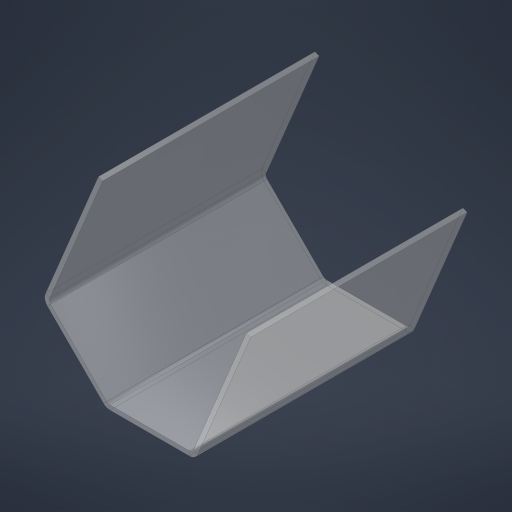
# Autodesk Inventor part: GP3-002
Saved by Autodesk Inventor 2023.4 (Build 274418000, 418)
## iProperties
Created: 2025-01-14
Part Number: GP3-002
Material: Polycarbonate, Clear
Document SubType Name: Sheet Metal
Designer: brand
Density: 1.2 g/cm^3
Sheet Metal Rule: Default
Appearance: Polycarbonate - Clear
Author: brand
Autodesk Inventor part; units mm, degrees
ref_plane "YZ Plane" through (0, 0, 0) normal (1, 0, 0) x (0, 1, 0)
ref_plane "XZ Plane" through (0, 0, 0) normal (0, 1, 0) x (-1, 0, 0)
ref_plane "XY Plane" through (0, 0, 0) normal (0, 0, 1) x (1, 0, 0)
sketch "Sketch1" plane through (0, 0, 0) normal (0, 1, 0) x (-1, 0, 0)
  line L0 (61.9125, 76.2) -> (-61.9125, 76.2)
  line L1 (-61.9125, 76.2) -> (-61.9125, -76.2)
  line L2 (-61.9125, -76.2) -> (61.9125, -76.2)
  line L3 (61.9125, -76.2) -> (61.9125, 76.2)
  line L4 (61.9125, 76.2) -> (-61.9125, -76.2) construction
  line L5 (-61.9125, 76.2) -> (61.9125, -76.2) construction
  point P0 (0, 0)
  dimension "d0" = 123.825
  dimension "d1" = 152.4
  measures "d0" distance of L1.end L2.end
  measures "d1" distance of L2.end L0.start
extrude "Plate1" add sketch "Sketch1" against normal blind 3.175
sketch "Sketch2" plane through (0, 0, 0) normal (0, 1, 0) x (1, 0, 0)
  line L0 (-61.9125, -76.2) -> (61.9125, -76.2) construction
  line L1 (0, -76.2) -> (0, 76.2)
  line L2 (61.9125, 76.2) -> (-61.9125, 76.2) construction
  point P0 (0, 0)
  constraints: 2 end point, 2 midpoint, 1 vertical
fold "Fold1" angle 45 bend radius 3.175 thickness 3.175 k factor 0.44 line from (0, 0, 76.2) to (0, 0, -76.2) line at bend centre moving side (-1, 0, 0) folds toward (0, 1, 0)
sketch "Sketch3" plane through (58.9792, -1.96, -76.2) normal (0.9238795, -0.3826834, 0) x (0.3826834, 0.9238795, 0)
  line L0 (0, 152.4) -> (0, 0)
  line L1 (0, 0) -> (101.6, 0)
  line L2 (101.6, 0) -> (101.6, 152.4)
  line L3 (101.6, 152.4) -> (0, 152.4)
  constraints: 8 end point
edge flange "Flange1" height 101.6 angle 67.5 thickness 3.175 bend radius 3.175 thickness toward (0.9238795, -0.3826834, 0) relief straight relief width 3.175 relief depth 1.5875 edges at (61.9125, 0, 0) wall of the first edge with corners at (58.9792, -1.96, 76.2) (58.9792, -1.96, -76.2) (97.8598, 91.9062, -76.2) (97.8598, 91.9062, 76.2)
bend "Bend1"
corner "Corner1"
sketch "Sketch4" plane through (-42.2706, 39.979, -76.2) normal (-0.9238795, 0.3826834, 0) x (0.3826834, 0.9238795, 0)
  line L0 (0, 152.4) -> (0, 0)
  line L1 (0, 0) -> (101.6, 0)
  line L2 (101.6, 0) -> (101.6, 152.4)
  line L3 (101.6, 152.4) -> (0, 152.4)
  constraints: 6 end point, 1 horizontal, 1 perpendicular, 1 vertical
edge flange "Flange2" height 101.6 angle 67.5 thickness 3.175 bend radius 3.175 thickness toward (-0.9238795, 0.3826834, 0) relief straight relief width 3.175 relief depth 1.5875 edges at (-45.2039, 41.1941, 0) wall of the first edge with corners at (-42.2706, 39.979, 76.2) (-42.2706, 39.979, -76.2) (-3.3899, 133.8452, -76.2) (-3.3899, 133.8452, 76.2)
bend "Bend2"
corner "Corner2"
equation "\"d2\" = Thickness"
equation "\"d3\" = BendReliefWidth"
equation "\"d4\" = BendReliefDepth"
equation "\"d5\" = MinimumRemnant"
equation "\"d6\" = TransitionRadius"
equation "\"d8\" = BendRadius"
equation "\"d9\" = BendReliefWidth"
equation "\"d10\" = BendReliefDepth"
equation "\"d11\" = MinimumRemnant"
equation "\"d12\" = TransitionRadius"
equation "\"d15\" = BendRadius"
equation "\"d16\" = CornerReliefSize"
equation "\"d17\" = GapSize"
equation "\"d18\" = JacobiRadiusSize"
equation "\"d19\" = BendReliefWidth"
equation "\"d20\" = BendReliefDepth"
equation "\"d21\" = MinimumRemnant"
equation "\"d22\" = TransitionRadius"
equation "\"d23\" = d13"
equation "\"d25\" = BendRadius"
equation "\"d26\" = CornerReliefSize"
equation "\"d27\" = GapSize"
equation "\"d28\" = JacobiRadiusSize"
equation "\"BendRadius\" = Thickness"
equation "\"BendReliefWidth\" = Thickness"
equation "\"BendReliefDepth\" = 0.5 * Thickness"
equation "\"CornerReliefSize\" = 4 * Thickness"
equation "\"MinimumRemnant\" = 2 * Thickness"
equation "\"TransitionRadius\" = BendRadius"
equation "\"JacobiRadiusSize\" = BendRadius"
equation "\"GapSize\" = Thickness"
equation "\"Thickness\" = 3.175"
equation "\"d13\" = 101.6"
body "Solid1"
